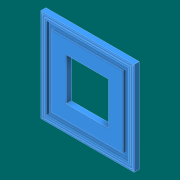
# Autodesk Inventor part: back
Saved by Autodesk Inventor 2016 (Build 200138000, 138)
## iProperties
Created: 2015-10-13
Part Number: back
Material: PC/ABS Plastic
Document SubType Name: Modeling
Designer: Sawaiz
Density: 0.357273 g/cm^3
Appearance: Cyan
Author: Sawaiz
Autodesk Inventor part; units mm, degrees
ref_plane "YZ Plane" through (0, 0, 0) normal (1, 0, 0) x (0, 1, 0)
ref_plane "XZ Plane" through (0, 0, 0) normal (0, 1, 0) x (-1, 0, 0)
ref_plane "XY Plane" through (0, 0, 0) normal (0, 0, 1) x (1, 0, 0)
sketch "Sketch1" plane through (0, 0, 0) normal (1, 0, 0) x (0, 1, 0)
  line L0 (-57.15, -57.15) -> (57.15, -57.15)
  line L1 (57.15, -57.15) -> (57.15, 57.15)
  line L2 (57.15, 57.15) -> (-57.15, 57.15)
  line L3 (-57.15, 57.15) -> (-57.15, -57.15)
  line L4 (-57.15, -57.15) -> (57.15, 57.15) construction
  line L5 (57.15, -57.15) -> (-57.15, 57.15) construction
  point P0 (0, 0)
  dimension "d0" = 114.3
  dimension "d1" = 114.3
  constraints: 12 end point, 2 midpoint, 2 parallel, 1 horizontal, 1 perpendicular
  measures "d0" distance of L2.end L1.end
  measures "d1" distance of L1.end L0.end
extrude "Extrusion1" add sketch "Sketch1" along normal blind 6.35
sketch "Sketch2" plane through (6.35, 0, 0) normal (1, 0, 0) x (0, 0, -1)
  line L0 (-26, 26) -> (26, 26)
  line L1 (26, 26) -> (26, -26)
  line L2 (26, -26) -> (-26, -26)
  line L3 (-26, -26) -> (-26, 26)
  line L4 (-26, 26) -> (26, -26) construction
  line L5 (26, 26) -> (-26, -26) construction
  point P0 (0, 0)
  dimension "d4" = 52
  dimension "d5" = 52
  constraints: 12 end point, 2 midpoint, 2 parallel, 1 horizontal, 1 perpendicular
  measures "d4" distance of L1.end L2.end
  measures "d5" distance of L0.end L1.end
extrude "Extrusion2" cut sketch "Sketch2" against normal through all
sketch "Sketch3" plane through (6.35, 0, 0) normal (1, 0, 0) x (0, 0, -1)
  line L0 (-26, -26) -> (-26, 26) projected
  line L1 (-26, 26) -> (26, 26) projected
  line L2 (26, 26) -> (26, -26) projected
  line L3 (26, -26) -> (-26, -26) projected
  line L4 (57.15, -57.15) -> (57.15, 57.15) projected
  line L5 (57.15, 57.15) -> (-57.15, 57.15) projected
  line L6 (-57.15, 57.15) -> (-57.15, -57.15) projected
  line L7 (-57.15, -57.15) -> (57.15, -57.15) projected
  line L8 (-57.15, -57.15) -> (57.15, -57.15) projected
  line L9 (43.803, -43.803) -> (-43.803, -43.803)
  line L10 (-43.803, -43.803) -> (-43.803, 43.803)
  line L11 (-43.803, 43.803) -> (43.803, 43.803)
  line L12 (43.803, 43.803) -> (43.803, -43.803)
  line L13 (43.803, -43.803) -> (-43.803, 43.803) construction
  line L14 (-43.803, -43.803) -> (43.803, 43.803) construction
  line L15 (-50.153, 50.153) -> (-50.153, -50.153)
  line L16 (-50.153, -50.153) -> (50.153, -50.153)
  line L17 (50.153, -50.153) -> (50.153, 50.153)
  line L18 (50.153, 50.153) -> (-50.153, 50.153)
  point P0 (0, 0)
  point P1 (0, 0)
  point P2 (0, 0)
  dimension "d92" = 13.347
  dimension "d93" = 13.347
  dimension "d94" = 6.35
  constraints: 20 end point, 4 parallel, 3 midpoint, 2 perpendicular, 1 coincident, 1 horizontal, 4 other
  measures "d92" distance between parallel lines of L10 L6
  measures "d93" distance between parallel lines of L7 L9
  measures "d94" distance between parallel lines of L10 L15
extrude "Extrusion3" cut sketch "Sketch3" against normal blind 3.175 contours L18 L17 L16 L15
sketch "Sketch4" plane through (0, 0, 0) normal (-1, 0, 0) x (0, 0, 1)
  line L0 (26, 26) -> (26, -26) projected
  line L1 (26, -26) -> (-26, -26) projected
  line L2 (-26, -26) -> (-26, 26) projected
  line L3 (-26, 26) -> (26, 26) projected
  line L4 (-57.15, -57.15) -> (-57.15, 57.15) projected
  line L5 (57.15, -57.15) -> (-57.15, -57.15) projected
  line L6 (57.15, 57.15) -> (57.15, -57.15) projected
  line L7 (-57.15, 57.15) -> (57.15, 57.15) projected
  line L8 (57.15, 57.15) -> (57.15, -57.15) projected
  line L9 (-57.15, 57.15) -> (57.15, 57.15) projected
  line L10 (-55.5625, 55.5625) -> (55.5625, 55.5625)
  line L11 (55.5625, 55.5625) -> (55.5625, -55.5625)
  line L12 (55.5625, -55.5625) -> (-55.5625, -55.5625)
  line L13 (-55.5625, -55.5625) -> (-55.5625, 55.5625)
  line L14 (-55.5625, 55.5625) -> (55.5625, -55.5625) construction
  line L15 (55.5625, 55.5625) -> (-55.5625, -55.5625) construction
  point P0 (0, 0)
  dimension "d83" = 1.5875
  dimension "d84" = 1.5875
  constraints: 12 end point, 4 coincident, 2 midpoint, 2 parallel, 1 horizontal, 1 perpendicular
  measures "d83" distance between parallel lines of L7 L10
  measures "d84" distance between parallel lines of L6 L11
hole "Hole1" at (0, 55.5625, 55.5625) at (0, 55.5625, -55.5625) at (0, -55.5625, -55.5625) at (0, -55.5625, 55.5625) direction (1, 0, 0) diameter 1.613 end through all countersink diameter 3.023 countersink angle 82 clearance for "Flat Head Machine Screw (82)" size "#0" standard "Ansi Unified Screw Threads"
sketch "Sketch6" plane through (6.35, 0, 0) normal (1, 0, 0) x (0, 0, -1)
  line L0 (57.15, -57.15) -> (57.15, 57.15) projected
  line L1 (57.15, 57.15) -> (-57.15, 57.15) projected
  line L2 (-57.15, 57.15) -> (-57.15, -57.15) projected
  line L3 (-57.15, -57.15) -> (57.15, -57.15) projected
  line L4 (52.3875, -52.3875) -> (-52.3875, -52.3875)
  line L5 (-52.3875, -52.3875) -> (-52.3875, 52.3875)
  line L6 (-52.3875, 52.3875) -> (52.3875, 52.3875)
  line L7 (52.3875, 52.3875) -> (52.3875, -52.3875)
  line L8 (52.3875, -52.3875) -> (-52.3875, 52.3875) construction
  line L9 (-52.3875, -52.3875) -> (52.3875, 52.3875) construction
  line L10 (-55.5625, 52.3875) -> (-55.5625, -52.3875)
  line L11 (-52.3875, -55.5625) -> (52.3875, -55.5625)
  line L12 (55.5625, -52.3875) -> (55.5625, 52.3875)
  line L13 (52.3875, 55.5625) -> (-52.3875, 55.5625)
  arc A0 (-55.5625, -52.3875) -> (-52.3875, -55.5625) centre (-52.3875, -52.3875) ccw
  arc A1 (-52.3875, 55.5625) -> (-55.5625, 52.3875) centre (-52.3875, 52.3875) ccw
  arc A2 (55.5625, 52.3875) -> (52.3875, 55.5625) centre (52.3875, 52.3875) ccw
  arc A3 (52.3875, -55.5625) -> (55.5625, -52.3875) centre (52.3875, -52.3875) ccw
  point P0 (0, 0)
  dimension "d88" = 104.775
  dimension "d89" = 104.775
  dimension "d90" = 3.175
  dimension "d91" = 3.175
  constraints: 20 end point, 8 point on circle, 8 tangent, 4 centre point, 4 parallel, 3 equal radius, 2 midpoint, 2 perpendicular, 1 horizontal, 3 other
  measures "d88" distance of L5.end L6.end
  measures "d89" distance of L4.end L5.end
  measures "d90" distance between parallel lines of L5 L10
  measures "d91" radius of A0
extrude "Extrusion4" cut sketch "Sketch6" against normal blind 0.9525 contours A1 L13 A2 L12 A3 L11 A0 L10
sketch "Sketch7" plane through (0, 0, 0) normal (-1, 0, 0) x (0, 0, 1)
  line L0 (26, 26) -> (26, -26) projected
  line L1 (26, -26) -> (-26, -26) projected
  line L2 (-26, -26) -> (-26, 26) projected
  line L3 (-26, 26) -> (26, 26) projected
  line L4 (-57.15, -57.15) -> (-57.15, 57.15) projected
  line L5 (57.15, -57.15) -> (-57.15, -57.15) projected
  line L6 (57.15, 57.15) -> (57.15, -57.15) projected
  line L7 (-57.15, 57.15) -> (57.15, 57.15) projected
  point P0 (0, 0)
  point P1 (55.5625, 55.5625)
  dimension "d74" = 1.5875
  dimension "d75" = 1.5875
  measures "d74" distance from line of L6 point (55.562, 55.562)
  measures "d75" distance from line of L7 point (55.562, 55.562)
hole "Hole3" at (0, 55.5625, 55.5625) direction (1, 0, 0) diameter 1.778 end through all countersink diameter 3.023 countersink angle 82 clearance for "Flat Head Machine Screw (82)" size "#0" standard "Ansi Unified Screw Threads"
sketch "Sketch8" plane through (0, 0, 0) normal (-1, 0, 0) x (0, 0, 1)
  line L0 (-44.45, 44.45) -> (44.45, 44.45)
  line L1 (44.45, 44.45) -> (44.45, -44.45)
  line L2 (44.45, -44.45) -> (-44.45, -44.45)
  line L3 (-44.45, -44.45) -> (-44.45, 44.45)
  line L4 (-44.45, 44.45) -> (44.45, -44.45) construction
  line L5 (44.45, 44.45) -> (-44.45, -44.45) construction
  line L6 (38.1, -38.1) -> (38.1, 38.1)
  line L7 (38.1, 38.1) -> (-38.1, 38.1)
  line L8 (-38.1, 38.1) -> (-38.1, -38.1)
  line L9 (-38.1, -38.1) -> (38.1, -38.1)
  line L10 (26, 26) -> (26, -26) projected
  line L11 (-26.9875, 26.9875) -> (26.9875, 26.9875)
  line L12 (26.9875, 26.9875) -> (26.9875, -26.9875)
  line L13 (26.9875, -26.9875) -> (-26.9875, -26.9875)
  line L14 (-26.9875, -26.9875) -> (-26.9875, 26.9875)
  line L15 (-26.9875, 26.9875) -> (26.9875, -26.9875) construction
  line L16 (26.9875, 26.9875) -> (-26.9875, -26.9875) construction
  point P0 (0, 0)
  point P1 (38.1, 20.6375)
  point P2 (-20.6375, 38.1)
  point P3 (-38.1, -20.6375)
  point P4 (20.6375, -38.1)
  dimension "d95" = 88.9
  dimension "d96" = 88.9
  dimension "d97" = 6.35
  dimension "d99" = 53.975
  dimension "d100" = 53.975
  dimension "d101" = 6.35
  dimension "d102" = 6.35
  dimension "d103" = 6.35
  dimension "d104" = 6.35
  constraints: 32 end point, 6 parallel, 4 coincident, 4 midpoint, 4 point on line, 3 perpendicular, 2 horizontal, 3 other
  measures "d95" distance of L1.end L2.end
  measures "d96" distance of L0.end L1.end
  measures "d97" distance between parallel lines of L0 L7
  measures "d99" distance of L12.end L13.end
  measures "d100" distance of L11.end L12.end
  measures "d101" distance from line of L12 point (20.638, -38.1)
  measures "d102" distance from line of L11 point (38.1, 20.637)
  measures "d103" distance from line of L14 point (-20.638, 38.1)
  measures "d104" distance from line of L13 point (-38.1, -20.637)
hole "Hole4" at (0, 38.1, 38.1) at (0, 38.1, -38.1) at (0, -38.1, -38.1) at (0, -38.1, 38.1) at (0, 20.6375, 38.1) at (0, 38.1, -20.6375) at (0, -20.6375, -38.1) at (0, -38.1, 20.6375) direction (1, 0, 0) diameter 1.181 depth 4.7625 tip angle 118 thread size "0-80 UNF" class "2B" standard "ANSI Unified Screw Threads"
equation "\"d0\" = height + 2 * acrylicThickness"
equation "\"d1\" = height + 2 * acrylicThickness"
equation "\"d2\" = acrylicThickness"
equation "\"d4\" = detectorHeight"
equation "\"d5\" = detectorWidth"
equation "\"d94\" = backMirrorGroove"
equation "\"d10\" = 0.5 * acrylicThickness"
equation "\"d83\" = 0.25 * acrylicThickness"
equation "\"d84\" = 0.25 * acrylicThickness"
equation "\"d88\" = 0.25 * frontBackORingID"
equation "\"d89\" = 0.25 * frontBackORingID"
equation "\"d90\" = oRingWidth"
equation "\"d91\" = oRingWidth"
equation "\"d74\" = 0.25 * acrylicThickness"
equation "\"d75\" = 0.25 * acrylicThickness"
equation "\"acrylicThickness\" = 6.35"
equation "\"height\" = 101.6"
equation "\"width\" = 101.6"
equation "\"depth\" = 101.6"
equation "\"mirrorAngle\" = 5deg"
equation "\"detectorWidth\" = 52"
equation "\"detectorHeight\" = 52"
equation "\"mirrorThickness\" = 3"
equation "\"fresnelThickness\" = 0.1"
equation "\"ior\" = 1.49"
equation "\"focalLength\" = 76.2"
equation "\"fresnelAngle\" = 90deg"
equation "\"centerThickness\" = 1.524"
equation "\"fresnelEffectiveDiameter\" = 76.2"
equation "\"mirrorSuppourtWidth\" = 38.1"
equation "\"backGrooveBit\" = 4.8006"
equation "\"sensorHolderHeight\" = 88.9"
equation "\"sensorHolderWidth\" = 88.9"
equation "\"sensorHolderSensorWidth\" = 53.975"
equation "\"sensorHolderSesnorHeight\" = 53.975"
equation "\"sensorHolderSensorHeight\" = 53.975"
equation "\"sensorHolderORingGroove\" = 3.175"
equation "\"sensorHolderORing\" = 3.175"
equation "\"sensorHolderFlushORingID\" = 254"
equation "\"sensorHolderFlushORing\" = 3.175"
equation "\"sensorHolderORingID\" = 203.2"
equation "\"oRingWidth\" = 3.175"
equation "\"frontBackORingID\" = 419.1"
equation "\"topBottomHorizontalMirrorGroove\" = 12.7"
equation "\"backMirrorGroove\" = 6.35"
equation "\"mirrorGroove\" = 19.05"
equation "\"fresnelChamfer\" = 6.35"
equation "\"mirrorGrooveFillet\" = 6.35"
equation "\"mirrorGrooveDrill\" = 6.35"
equation "\"mirrorGrooveMill\" = 3.175"
body "Solid1"
